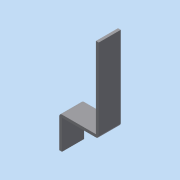
# Autodesk Inventor part: Crystal_L_Strip
Saved by Autodesk Inventor 2014 (Build 180170000, 170)
## iProperties
Created: 2014-04-18
Part Number: Crystal_L_Strip
Material: Generic
Document SubType Name: Sheet Metal
Designer: RDavis
Density: 1 g/cm^3
Sheet Metal Rule: Default_mm
Appearance: Default
Flat Pattern Width: 0.3 cm
Flat Pattern Length: 2.0146 cm
Flat Pattern Area: 0.60438 cm^2
Sheet Metal Width: 3.000 mm
Sheet Metal Length: 20.146 mm
Sheet Metal Area: 60.438 mm^2
Author: RDavis
Autodesk Inventor part; units mm, degrees
ref_plane "YZ Plane" through (0, 0, 0) normal (1, 0, 0) x (0, 1, 0)
ref_plane "XZ Plane" through (0, 0, 0) normal (0, 1, 0) x (-1, 0, 0)
ref_plane "XY Plane" through (0, 0, 0) normal (0, 0, 1) x (1, 0, 0)
sketch "Sketch1" plane through (0, 0, 0) normal (0, 0, 1) x (1, 0, 0)
  line L0 (-10.073, 1.5) -> (10.073, 1.5)
  line L1 (10.073, 1.5) -> (10.073, -1.5)
  line L2 (10.073, -1.5) -> (-10.073, -1.5)
  line L3 (-10.073, -1.5) -> (-10.073, 1.5)
  line L4 (0, 0) -> (0, 1.1953)
  line L5 (0, 0) -> (1.5725, 0)
  dimension "d0" = 20.146
  dimension "d1" = 3
  measures "d0" distance of L0.start L0.end
  measures "d1" distance of L0.end L1.end
extrude "Plate1" add sketch "Sketch1" along normal blind 0.381
sketch "Sketch2" plane through (0, 0, 0.381) normal (0, 0, 1) x (1, 0, 0)
  line L0 (-10.073, 1.5) -> (10.073, 1.5) projected
  line L1 (10.073, -1.5) -> (-10.073, -1.5) projected
  line L2 (-1.059, 1.5) -> (-1.059, -1.5)
  line L3 (10.073, 1.5) -> (10.073, -1.5) projected
  point P0 (0, 0)
  dimension "d10" = 11.132
  constraints: 2 end point, 2 point on line, 1 vertical
  measures "d10" distance between parallel lines of L3 L2
fold "Fold1" angle 90 bend radius 0.001 thickness 0.381 k factor 0.44 line from (-1.059, 1.5, 0.381) to (-1.059, -1.5, 0.381) line at bend centre moving side (1, 0, 0) folds toward (0, 0, 1)
sketch "Sketch4" plane through (0, 0, 0.381) normal (0, 0, 1) x (1, 0, 0)
  line L0 (-10.073, 1.5) -> (-1.1914, 1.5) projected
  line L1 (-10.073, -1.5) -> (-10.073, 1.5) projected
  line L2 (-1.1914, -1.5) -> (-10.073, -1.5) projected
  line L3 (-5.941, 1.5) -> (-5.941, -1.5)
  point P0 (0, 0)
  dimension "d11" = 4.132
  constraints: 2 end point, 2 point on line, 1 vertical
  measures "d11" distance between parallel lines of L3 L1
fold "Fold2" angle 90 bend radius 0.001 thickness 0.381 k factor 0.44 line from (-5.941, 1.5, 0.381) to (-5.941, -1.5, 0.381) line at bend centre moving side (-1, 0, 0) folds toward (0, 0, -1)
equation "\"d4\" = BendReliefWidth"
equation "\"d5\" = BendReliefDepth"
equation "\"d6\" = MinimumRemnant"
equation "\"d7\" = BendRadius"
equation "\"d9\" = BendRadius"
equation "\"d12\" = BendReliefWidth"
equation "\"d13\" = BendReliefDepth"
equation "\"d14\" = MinimumRemnant"
equation "\"d15\" = BendRadius"
equation "\"d17\" = BendRadius"
equation "\"BendReliefWidth\" = Thickness"
equation "\"BendReliefDepth\" = 0.5 * Thickness"
equation "\"CornerReliefSize\" = 4 * Thickness"
equation "\"MinimumRemnant\" = 2 * Thickness"
equation "\"TransitionRadius\" = BendRadius"
equation "\"JacobiRadiusSize\" = BendRadius"
equation "\"GapSize\" = Thickness"
equation "\"d2\" = BendRadius"
equation "\"BendRadius\" = 0.001"
equation "\"Thickness\" = 0.381"
body "Solid1"
